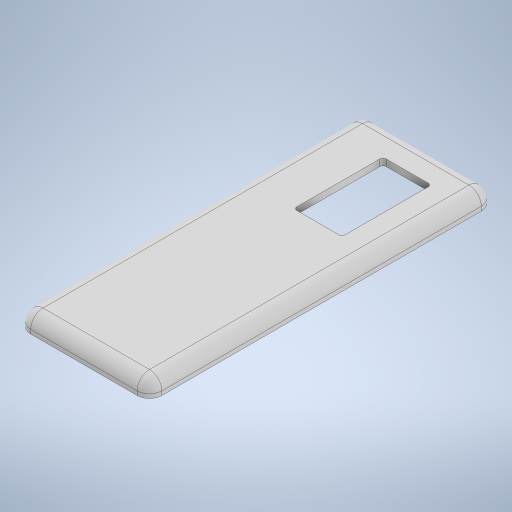
# Autodesk Inventor part: LI0002-CASE LID
Saved by Autodesk Inventor 2023 (Build 270158000, 158)
## iProperties
Created: 2023-03-14
Part Number: LI0002-CASE LID
Material: Generic
Document SubType Name: Modeling
Designer: Louis
Density: 1 g/cm^3
Appearance: Default
Mass: 342.382 g
Surface Area: 778.94 cm^2
Volume: 342.382 cm^3
Author: Louis
Autodesk Inventor part; units mm, degrees
ref_plane "YZ Plane" through (0, 0, 0) normal (1, 0, 0) x (0, 1, 0)
ref_plane "XZ Plane" through (0, 0, 0) normal (0, 1, 0) x (-1, 0, 0)
sketch "Sketch1" plane through (0, 0, 0) normal (0, 1, 0) x (-1, 0, 0)
  line L0 (80, 210) -> (-80, 210)
  line L1 (-80, 210) -> (-80, -210)
  line L2 (-80, -210) -> (80, -210)
  line L3 (80, -210) -> (80, 210)
  point P0 (0, 0)
  point P1 (80, 0)
  point P2 (0, -210)
  dimension "d1" = 420
  dimension "d2" = 160
  constraints: 8 end point, 2 midpoint, 2 parallel, 1 horizontal, 1 horizontal alignment, 1 perpendicular, 1 vertical alignment
  measures "d1" distance of L2.end L0.start
  measures "d2" distance of L1.end L2.end
extrude "Extrusion1" add sketch "Sketch1" along normal blind 20
shell "Shell1" thickness 10 removed faces 1 at (-26.6667, 0, -70)
sketch "Sketch2" plane through (0, 0, 0) normal (0, -1, 0) x (1, 0, 0)
  line L0 (80, -210) -> (-80, -210) projected
  line L1 (-80, -210) -> (-57, -210)
  line L2 (-57, -210) -> (-57, -187)
  line L3 (-57, -187) -> (-80, -187)
  line L4 (-80, -187) -> (-80, -210)
  line L5 (-80, -210) -> (-80, 210) projected
  line L6 (-80, 210) -> (-57, 210)
  line L7 (-57, 210) -> (-57, 187)
  line L8 (-57, 187) -> (-80, 187)
  line L9 (-80, 187) -> (-80, 210)
  line L10 (-80, 210) -> (80, 210) projected
  line L11 (80, 210) -> (57, 210)
  line L12 (57, 210) -> (57, 187)
  line L13 (57, 187) -> (80, 187)
  line L14 (80, 187) -> (80, 210)
  line L15 (80, -210) -> (57, -210)
  line L16 (57, -210) -> (57, -187)
  line L17 (57, -187) -> (80, -187)
  line L18 (80, -187) -> (80, -210)
  point P0 (0, 0)
  point P1 (-80, 187)
  point P2 (57, -210)
  dimension "d6" = 23
  constraints: 32 end point, 8 parallel, 7 perpendicular, 6 point on line, 4 horizontal
  measures "d6" distance of L2.end L3.end
extrude "Extrusion2" add sketch "Sketch2" against normal up to surface (10 mm away)
sketch "Sketch3" plane through (0, 0, 0) normal (0, -1, 0) x (1, 0, 0)
  line L0 (-57, -187) -> (-70, -187) projected
  line L1 (-57, -200) -> (-57, -187) projected
  line L2 (57, 200) -> (57, 187) projected
  line L3 (57, 187) -> (70, 187) projected
  line L4 (80, 210) -> (80, -210) projected
  line L5 (-80, 210) -> (80, 210) projected
  line L6 (80, -210) -> (-80, -210) projected
  line L7 (-80, -210) -> (-80, 210) projected
  point P0 (0, 0)
  point P1 (-65, -195)
  point P2 (-65, 195)
  point P3 (65, -195)
  point P4 (65, 195)
  dimension "d22" = 15
  dimension "d23" = 15
  dimension "d24" = 15
  dimension "d25" = 15
  constraints: 2 horizontal alignment, 2 vertical alignment
  measures "d22" distance from line of L4 point (65, 195)
  measures "d23" distance from line of L5 point (65, 195)
  measures "d24" distance from line of L6 point (-65, -195)
  measures "d25" distance from line of L7 point (-65, -195)
hole "Hole1" at (-65, 0, -195) at (-65, 0, 195) at (65, 0, -195) at (65, 0, 195) direction (0, 1, 0) diameter 10.1 depth 10
sketch "Sketch7" plane through (-57, 10, -200) normal (0, -1, 0) x (1, 0, 0)
  line L0 (-13, 13) -> (-13, 387) projected
  line L1 (127, 387) -> (127, 13) projected
  line L2 (-13, 260) -> (127, 260)
  line L3 (127, 260) -> (127, 265)
  line L4 (127, 265) -> (-13, 265)
  line L5 (-13, 265) -> (-13, 260)
  line L6 (0, 400) -> (114, 400) projected
  line L7 (-23, 410) -> (137, 410) projected
  point P0 (-13, 262.5)
  point P1 (-13, 265)
  point P2 (127, 260)
  dimension "d51" = 5
  dimension "d89" = 145
  constraints: 8 end point, 2 parallel, 2 point on line, 1 horizontal, 1 midpoint, 1 perpendicular
  measures "d51" distance between parallel lines of L4 L2
  measures "d89" distance between parallel lines of L4 L7
extrude "Extrusion5" add sketch "Sketch7" along normal up to surface (10 mm away)
fillet "Fillet1" radius 15 8 edges at (-80, 10, -210) (-80, 20, 0) (0, 20, -210) (80, 20, 0) (80, 10, -210) (80, 10, 210) (0, 20, 210) (-80, 10, 210)
fillet "Fillet2" radius 5 32 edges at (70, 5, 187) (57, 5, 187) (57, 5, 200) (-57, 5, 200) (-57, 5, 187) (-70, 5, 187) (-70, 5, -187) (-57, 5, -187) (-57, 5, -200) (57, 5, -200) (57, 5, -187) (70, 5, -187) (0, 10, 200) (70, 10, -63.5) (70, 10, 126) (63.5, 10, 187) (57, 10, 193.5) (-57, 10, 193.5) (-63.5, 10, 187) (-70, 10, -63.5) (-70, 10, 126) (-63.5, 10, -187) (-57, 10, -193.5) (0, 10, -200) (57, 10, -193.5) (63.5, 10, -187) (-70, 5, 60) (-70, 5, 65) (0, 10, 65) (0, 10, 60) (70, 5, 65) (70, 5, 60)
sketch "Sketch4" plane through (0, 0, 0) normal (0, -1, 0) x (1, 0, 0)
  line L0 (80, 195) -> (80, -195) projected
  arc A0 (80, 195) -> (65, 210) centre (65, 195) ccw projected
  line L1 (-65, 210) -> (65, 210) projected
  arc A1 (-65, 210) -> (-80, 195) centre (-65, 195) ccw projected
  line L2 (-80, -195) -> (-80, 195) projected
  arc A2 (-80, -195) -> (-65, -210) centre (-65, -195) ccw projected
  line L3 (65, -210) -> (-65, -210) projected
  arc A3 (65, -210) -> (80, -195) centre (65, -195) ccw projected
  line L4 (77, -195) -> (77, 195)
  arc A4 (77, 195) -> (65, 207) centre (65, 195) ccw
  line L5 (65, 207) -> (-65, 207)
  arc A5 (-65, 207) -> (-77, 195) centre (-65, 195) ccw
  line L6 (-77, 195) -> (-77, -195)
  arc A6 (-77, -195) -> (-65, -207) centre (-65, -195) ccw
  line L7 (-65, -207) -> (65, -207)
  arc A7 (65, -207) -> (77, -195) centre (65, -195) ccw
  line L8 (73, -195) -> (73, 195)
  arc A8 (73, 195) -> (65, 203) centre (65, 195) ccw
  line L9 (65, 203) -> (-65, 203)
  arc A9 (-65, 203) -> (-73, 195) centre (-65, 195) ccw
  line L10 (-73, 195) -> (-73, -195)
  arc A10 (-73, -195) -> (-65, -203) centre (-65, -195) ccw
  line L11 (-65, -203) -> (65, -203)
  arc A11 (65, -203) -> (73, -195) centre (65, -195) ccw
  point P0 (0, 0)
  point P1 (75, 150)
  point P2 (75, -150)
  point P3 (-75, 150)
  point P4 (-75, -150)
  dimension "d26" = 3
  dimension "d27" = 7
  constraints: 16 end point, 16 point on circle, 8 centre point, 18 other
extrude "Extrusion3" cut sketch "Sketch4" against normal blind 2 contours A7 L7 A6 L6 A5 L5 A4 L4
chamfer "Chamfer1" distance 0.5 angle 45 16 edges at (0, 0, 203) (-70.6569, 0, 200.6569) (-73, 0, 0) (-70.6569, 0, -200.6569) (0, 0, -203) (70.6569, 0, -200.6569) (73, 0, 0) (70.6569, 0, 200.6569) (0, 0, 207) (73.4853, 0, 203.4853) (77, 0, 0) (73.4853, 0, -203.4853) (0, 0, -207) (-73.4853, 0, -203.4853) (-77, 0, 0) (-73.4853, 0, 203.4853)
chamfer "Chamfer2" distance 1 angle 60 1 edges at (65, 0, 200.05) measured on face at (65, 0, 200.55)
chamfer "Chamfer3" distance 1 angle 60 1 edges at (-65, 0, 200.05) measured on face at (-65, 0, 200.55)
chamfer "Chamfer4" distance 1 angle 60 1 edges at (-65, 0, -189.95) measured on face at (-65, 0, -189.45)
chamfer "Chamfer5" distance 1 angle 60 1 edges at (65, 0, -189.95) measured on face at (65, 0, -189.45)
sketch "Sketch15" plane through (-52, 10, -195) normal (0, -1, 0) x (1, 0, 0)
  line L0 (102, 140) -> (27, 140)
  line L1 (27, 140) -> (27, 15)
  line L2 (27, 15) -> (102, 15)
  line L3 (102, 15) -> (102, 140)
  line L4 (117, 250) -> (117, 13) projected
  line L5 (104, 0) -> (0, 0) projected
  line L6 (88, 150) -> (86, 150) projected
  point P0 (52, 195)
  dimension "d99" = 15
  dimension "d100" = 15
  dimension "d101" = 10
  dimension "d207" = 75
  constraints: 8 end point, 2 parallel, 1 horizontal, 1 perpendicular
  measures "d99" distance between parallel lines of L4 L3
  measures "d100" distance between parallel lines of L5 L2
  measures "d101" distance between parallel lines of L0 L6
  measures "d207" distance between parallel lines of L3 L1
extrude "Extrusion11" cut sketch "Sketch15" against normal blind 2
sketch "Sketch18" plane through (-52, 12, -195) normal (0, -1, 0) x (1, 0, 0)
  line L0 (102, 140) -> (102, 15) projected
  line L1 (27, 140) -> (102, 140) projected
  line L2 (27, 15) -> (27, 140) projected
  line L3 (102, 15) -> (27, 15) projected
  line L4 (35, 132) -> (94, 132)
  line L5 (94, 132) -> (94, 23)
  line L6 (94, 23) -> (35, 23)
  line L7 (35, 23) -> (35, 132)
  point P0 (52, 195)
  dimension "d115" = 8
  constraints: 8 end point, 3 other
  measures "d115" distance between parallel lines of L2 L7
extrude "Extrusion13" cut sketch "Sketch18" against normal through all contours L4 L5 L6 L7
sketch "Sketch19" plane through (-52, 12, -195) normal (0, -1, 0) x (1, 0, 0)
  line L0 (94, 132) -> (94, 23) projected
  line L1 (94, 23) -> (35, 23) projected
  line L2 (35, 23) -> (35, 132) projected
  line L3 (35, 132) -> (94, 132) projected
  line L4 (27, 15) -> (27, 140) projected
  line L5 (102, 15) -> (27, 15) projected
  line L6 (102, 140) -> (102, 15) projected
  line L7 (27, 140) -> (102, 140) projected
  line L8 (99, 18) -> (30, 18)
  line L9 (30, 18) -> (30, 137)
  line L10 (30, 137) -> (99, 137)
  line L11 (99, 137) -> (99, 18)
  point P0 (52, 195)
  dimension "d118" = 3
  constraints: 8 end point, 4 coincident, 3 other
  measures "d118" distance between parallel lines of L6 L11
hole "Hole3" at (47, 12, -58) at (47, 12, -177) at (-22, 12, -58) at (-22, 12, -177) direction (0, 1, 0) diameter 2.459 depth 6 tip angle 118 thread size "M3x0.5" class "6H" standard "ISO Metric profile"
sketch "Sketch20" plane through (-52, 12, -195) normal (0, -1, 0) x (1, 0, 0)
  line L0 (27, 140) -> (102, 140) projected
  circle A0 centre (30, 137) radius 1.2295 projected
  circle A1 centre (99, 137) radius 1.2295 projected
  circle A2 centre (99, 18) radius 1.2295 projected
  circle A3 centre (30, 18) radius 1.2295 projected
  line L1 (94, 132) -> (94, 23) projected
  line L2 (94, 23) -> (35, 23) projected
  line L3 (35, 23) -> (35, 132) projected
  line L4 (35, 132) -> (94, 132) projected
  line L5 (27, 15) -> (27, 140) projected
  line L6 (102, 15) -> (27, 15) projected
  line L7 (102, 140) -> (102, 15) projected
  line L8 (27, 140) -> (102, 140) projected
  line L9 (98, 19) -> (31, 19)
  line L10 (31, 19) -> (31, 136)
  line L11 (31, 136) -> (98, 136)
  line L12 (98, 136) -> (98, 19)
  line L13 (96, 21) -> (33, 21)
  line L14 (33, 21) -> (33, 134)
  line L15 (33, 134) -> (96, 134)
  line L16 (96, 134) -> (96, 21)
  point P0 (52, 195)
  dimension "d126" = 4
  dimension "d127" = 2
  constraints: 16 end point, 6 other
  measures "d126" distance between parallel lines of L7 L12
  measures "d127" distance between parallel lines of L12 L16
extrude "Extrusion14" cut sketch "Sketch20" against normal blind 2 contours L9 L10 L11 L12
fillet "Fillet5" radius 2 8 edges at (50, 11, -55) (-25, 11, -55) (-25, 11, -180) (50, 11, -180) (44, 13, -174) (-19, 13, -174) (-19, 13, -61) (44, 13, -61)
fillet "Fillet6" radius 4 4 edges at (-21, 13, -59) (46, 13, -59) (46, 13, -176) (-21, 13, -176)
fillet "Fillet7" radius 4 4 edges at (-17, 16, -63) (42, 16, -63) (42, 16, -172) (-17, 16, -172)
sketch "Sketch21" plane through (65, 0, 60) normal (0, 0, -1) x (-1, 0, 0)
  line L0 (0, 0) -> (130, 0) projected
  line L1 (24, 0) -> (9, 0)
  line L2 (9, 0) -> (9, 5)
  line L3 (9, 5) -> (24, 5)
  line L4 (24, 5) -> (24, 0)
  line L5 (-5, 5) -> (-5, 0) projected
  point P0 (65, 0)
  point P1 (26.8459, 10)
  point P2 (9, 0)
  dimension "d208" = 15
  dimension "d209" = 5
  dimension "d231" = 14
  constraints: 8 end point, 2 parallel, 1 horizontal, 1 perpendicular, 1 point on line
  measures "d208" distance of L2.end L3.end
  measures "d209" distance of L1.end L2.end
  measures "d231" distance between parallel lines of L5 L2
extrude "Extrusion15" cut sketch "Sketch21" against normal blind 10
fillet "Fillet8" radius 2 2 edges at (41, 5, 62.5) (56, 5, 62.5)
sketch "Sketch22" plane through (-65, 0, 60) normal (0, 0, -1) x (-1, 0, 0)
  line L0 (-106, 0) -> (0, 0) projected
  line L1 (-1, 0) -> (-5, 0)
  line L2 (-5, 0) -> (-5, 10)
  line L3 (-5, 10) -> (-1, 10)
  line L4 (-1, 10) -> (-1, 0)
  line L5 (0, 10) -> (-130, 10) projected
  line L6 (0, 5) -> (0, 0) projected
  line L7 (-1, 0) -> (1, 0)
  line L8 (1, 0) -> (1, 10)
  line L9 (1, 10) -> (-1, 10)
  line L10 (-1, 10) -> (-1, 0)
  line L11 (-5, 0) -> (-7, 0)
  line L12 (-7, 0) -> (-7, 10)
  line L13 (-7, 10) -> (-5, 10)
  line L14 (-5, 10) -> (-5, 0)
  line L15 (-7, 10) -> (-9, 10)
  line L16 (-9, 10) -> (-7, 0)
  line L17 (1, 10) -> (3, 10)
  line L18 (3, 10) -> (1, 0)
  point P0 (-65, 0)
  point P1 (-3, 0)
  point P2 (-1, 10)
  point P3 (0, 0)
  point P4 (-7, 10)
  point P5 (-5, 0)
  point P6 (-5, 10)
  dimension "d218" = 4
  dimension "d219" = 3
  dimension "d220" = 2
  dimension "d221" = 2
  dimension "d235" = 2
  dimension "d236" = 2
  constraints: 32 end point, 6 parallel, 3 collinear, 3 horizontal, 3 perpendicular, 3 point on line, 1 midpoint
  measures "d218" distance between parallel lines of L4 L2
  measures "d219" distance from line of L6 point (-3, 0)
  measures "d220" distance between parallel lines of L2 L12
  measures "d221" distance between parallel lines of L8 L4
  measures "d235" distance of L8.end L17.end
  measures "d236" distance of L12.end L15.end
extrude "Extrusion16" add sketch "Sketch22" along normal blind 100 contours L12 L5 L2 L0 | L16 L5 L12 | L4 L5 L9 L8 L7 L0 | L8 L17 L18
ref_plane "Work Plane6" through (-65, 0, 62.5) normal (0, 0, -1) x (-1, 0, 0)
mirror "Mirror5" about plane through (-65, 0, 62.5) normal (0, 0, -1) of "Extrusion16"
pattern_linear "Rectangular Pattern6" count 3 spacing 45 along (1, 0, 0) of "Extrusion16", "Mirror5"
thicken "Thicken38" operation add thickness 100 both sides no extend neighbours no toward (0, 0, -1) faces at (-58, 6.6667, -40)
thicken "Thicken39" operation add thickness 100 both sides no extend neighbours no toward (0, 0, -1) faces at (-65.6084, 6.3751, -40)
pattern_linear "Rectangular Pattern7" count 3 spacing 45 along (-1, 0, 0) of "Extrusion15", "Fillet8"
body "Solid1"
